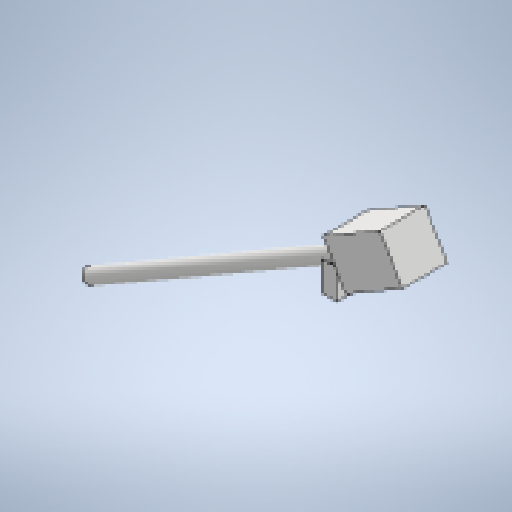
# Autodesk Inventor part: NDM-VOS dummy5
Saved by Autodesk Inventor 2025.1 (Build 291241020, 241B)
## iProperties
Created: 2024-10-01
Part Number: NDM-VOS dummy5
Material: Generic
Document SubType Name: Modeling
Designer: pokla
Density: 1 g/cm^3
Appearance: Default
Author: pokla
Autodesk Inventor part; units mm, degrees
ref_plane "YZ Plane" through (0, 0, 0) normal (1, 0, 0) x (0, 1, 0)
ref_plane "XZ Plane" through (0, 0, 0) normal (0, 1, 0) x (-1, 0, 0)
ref_plane "XY Plane" through (0, 0, 0) normal (0, 0, 1) x (1, 0, 0)
sketch "Sketch2" plane through (0, 0, 0) normal (0, 1, 0) x (-1, 0, 0)
  line L0 (1299.0381, 1500) -> (-433.0127, 2500)
  line L1 (1299.0381, 1500) -> (-700.9619, 1500) construction
  line L2 (0, 0) -> (0, 2250)
  line L3 (-358.0127, 2629.9038) -> (-791.0254, 2879.9038)
  line L4 (-791.0254, 2879.9038) -> (-941.0254, 2620.0962)
  line L5 (-941.0254, 2620.0962) -> (-508.0127, 2370.0962)
  line L6 (-508.0127, 2370.0962) -> (-358.0127, 2629.9038)
  line L7 (-409.9742, 2659.9038) -> (-559.9742, 2400.0962)
  line L8 (-447.4742, 2594.9519) -> (-395.5127, 2564.9519)
  line L9 (-522.4742, 2465.0481) -> (-470.5127, 2435.0481)
  line L10 (-303.1089, 2425) -> (-403.1089, 2425)
  line L11 (-403.1089, 2425) -> (-403.1089, 2225)
  line L12 (-403.1089, 2225) -> (-303.1089, 2225)
  line L13 (-303.1089, 2225) -> (-303.1089, 2425)
  line L14 (-303.1089, 2425) -> (-403.1089, 2225) construction
  line L15 (-403.1089, 2425) -> (-303.1089, 2225) construction
  point P0 (-353.1089, 2325)
  dimension "d3" = 30
  dimension "d4" = 2000
  dimension "d10" = 2250
  dimension "d11" = 500
  dimension "d12" = 500
  dimension "d13" = 300
  dimension "d14" = 150
  dimension "d15" = 60
  dimension "d16" = 100
  dimension "d17" = 200
  dimension "d18" = 150
  constraints: 32 end point, 8 point on line, 5 parallel, 5 perpendicular, 3 midpoint, 2 horizontal, 1 equal length, 1 vertical, 1 other
  measures "d3" angle of L1 L0
  measures "d4" distance of L0.end L0.start
  measures "d10" distance of L2.start L2.end
  measures "d11" distance of L0.end L2.end
  measures "d12" distance of L3.start L3.end
  measures "d13" distance of L5.end L3.start
  measures "d14" distance between parallel lines of L9 L8
  measures "d15" distance of L9.start L9.end
  measures "d16" distance of L11.end L12.end
  measures "d17" distance of L12.end L10.start
  measures "d18" distance of L10.start L0.end
ref_plane "Work Plane1" through (-1299.0381, 0, 1500) normal (0.866, 0, 0.5) x (0, 1, 0)
sketch "Sketch3" plane through (-1299.0381, 0, 1500) normal (0.866, 0, 0.5) x (0, 1, 0)
  circle A0 centre (0, 0) radius 50
  circle A1 centre (0, 0) radius 47
  point P0 (0, -1948.5572)
  point P1 (0, 0)
  dimension "d6" = 100
  dimension "d7" = 3
  constraints: 2 centre point, 1 coincident
  measures "d6" diameter of A0
  measures "d7" radial gap between concentric circles of A0 A1
sweep "Sweep1" add profiles "Sketch3" path "Sketch2" path curves L0
extrude "Extrusion2" add sketch "Sketch2" along normal mid plane 100 contours L6 L9 L7 L8 | L13 L12 L11 L10
extrude "Extrusion3" add sketch "Sketch2" along normal mid plane 300 contours L7 L5 L4 L3
equation "\"d16\" = d6"
equation "\"d19\" = d6"
body "Solid2"
